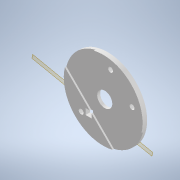
# Autodesk Inventor part: Matchboxscope_sample_v0
Saved by Autodesk Inventor 2022 (Build 260153000, 153)
## iProperties
Created: 2022-03-21
Part Number: Matchboxscope_sample_v0
Material: Generic
Document SubType Name: Modeling
Designer: Prakash Lab
Density: 1 g/cm^3
Appearance: Default
Author: Prakash Lab
Autodesk Inventor part; units mm, degrees
ref_plane "YZ Plane" through (0, 0, 0) normal (1, 0, 0) x (0, 1, 0)
ref_plane "XZ Plane" through (0, 0, 0) normal (0, 1, 0) x (-1, 0, 0)
ref_plane "XY Plane" through (0, 0, 0) normal (0, 0, 1) x (1, 0, 0)
ref_plane "Work Plane1" through (0, 0, 0) normal (0, 0, 1) x (0.9792327, -0.2027397, 0)
sketch "Sketch1" plane through (0, 0, 0) normal (0, 0, 1) x (0.9792327, -0.2027397, 0)
  circle A0 centre (8.0687, 11.3576) radius 25.9979 projected
  circle A1 centre (8.0703, 11.3562) radius 3.8103 projected
  circle A2 centre (8.0703, 11.3562) radius 5
  point P0 (0, 0)
  dimension "d0" = 10
  constraints: 1 centre point, 1 coincident
  measures "d0" diameter of A2
extrude "Extrusion1" add sketch "Sketch1" along normal blind 4 contours A0
sketch "Sketch2" plane through (10.2037, 9.4859, 4) normal (0, 0, 1) x (1, 0, 0)
  line L0 (-10.2037, 54.0449) -> (-10.2037, -50.593) projected
  line L1 (-54.0467, -9.4859) -> (50.5907, -9.4859) projected
  line L2 (-15.9479, -15.1669) -> (4.4725, 20.2023)
  line L3 (4.4725, 20.2023) -> (19.4213, 5.2535)
  line L4 (19.4213, 5.2535) -> (-15.9479, -15.1669)
  line L5 (-39.0985, 39.0967) -> (35.6425, -35.6447)
  line L6 (-0.781, 0) -> (9.2905, 10.0715)
  line L7 (-0.781, 0) -> (13.4622, 0) construction
  line L8 (-15.9479, -15.1669) -> (-0.781, 0)
  circle A0 centre (4.4725, 20.2023) radius 1.6
  circle A1 centre (19.4213, 5.2535) radius 1.6
  circle A2 centre (-15.9479, -15.1669) radius 1.6
  dimension "d17" = 18
  dimension "d18" = 22
  dimension "d19" = 30
  dimension "d20" = 45
  dimension "d21" = 15
  dimension "d22" = 3.2
  dimension "d23" = 3.2
  dimension "d24" = 3.2
  constraints: 14 end point, 3 centre point, 3 coincident, 1 collinear, 1 equal length, 1 horizontal, 1 parallel, 3 other
  measures "d17" distance from line of L6.start L3
  measures "d18" distance from line of L5 L2.start
  measures "d19" angle of L2 L4
  measures "d20" angle of L7 L6
  measures "d21" angle of L2 L6
  measures "d22" diameter of A0
  measures "d23" diameter of A1
  measures "d24" diameter of A2
extrude "Extrusion2" cut sketch "Sketch2" against normal through all contours A0 L3 L2 | L2 L3 A0 | A2 L8 L2 | L2 L4 A2 | A2 L4 L8 | A1 L4 L3 | L3 L4 A1
sketch "Sketch3" plane through (10.2037, 9.4859, 4) normal (0, 0, 1) x (1, 0, 0)
  line L0 (-35.7047, 22.4019) -> (13.1872, -35.1292) projected
  line L1 (32.542, -18.6808) -> (-16.3499, 38.8503) projected
  line L2 (40.2702, -21.1784) -> (-21.1782, 40.2703)
  line L3 (-21.1782, 40.2703) -> (-40.2702, 21.1784)
  line L4 (-40.2702, 21.1784) -> (21.1782, -40.2703)
  line L5 (21.1782, -40.2703) -> (40.2702, -21.1784)
  line L6 (40.2702, -21.1784) -> (-40.2702, 21.1784) construction
  line L7 (-21.1782, 40.2703) -> (21.1782, -40.2703) construction
  point P0 (0, 0)
  dimension "d16" = 27
  constraints: 12 end point, 2 midpoint, 2 parallel, 1 perpendicular
  measures "d16" distance of L3.end L2.end
extrude "Extrusion3" cut sketch "Sketch3" against normal blind 1
sketch "Sketch4" plane through (0, 0, 4) normal (0, 0, 1) x (0.9792327, -0.2027397, 0)
  circle A0 centre (-11.3769, -5.9318) radius 1.02 projected
  line L0 (-17.8452, -14.9951) -> (20.0302, -11.9207) projected
  line L1 (-7.3769, -9.6034) -> (-11.3769, -9.6034)
  line L2 (-11.3769, -9.6034) -> (-11.3769, -13.6034)
  line L3 (-11.3769, -13.6034) -> (-7.3769, -13.6034)
  line L4 (-7.3769, -13.6034) -> (-7.3769, -9.6034)
  line L5 (-7.3769, -9.6034) -> (-11.3769, -13.6034) construction
  line L6 (-11.3769, -9.6034) -> (-7.3769, -13.6034) construction
  circle A1 centre (-2.4923, 4.0739) radius 1 projected
  line L7 (-7.7982, -5.7154) -> (29.4127, 1.9886) projected
  line L8 (-1.2714, -1.0289) -> (2.6455, -0.218)
  line L9 (2.6455, -0.218) -> (3.4565, -4.1349)
  line L10 (3.4565, -4.1349) -> (-0.4605, -4.9459)
  line L11 (-0.4605, -4.9459) -> (-1.2714, -1.0289)
  line L12 (-1.2714, -1.0289) -> (3.4565, -4.1349) construction
  line L13 (2.6455, -0.218) -> (-0.4605, -4.9459) construction
  line L14 (-1.2714, -1.0289) -> (2.7286, -1.0289) construction
  point P0 (0, 0)
  point P1 (-9.3769, -11.6034)
  point P2 (1.0925, -2.5819)
  dimension "d25" = 2
  dimension "d28" = 4
  dimension "d29" = 4
  dimension "d30" = 4
  dimension "d31" = 11.697
  dimension "d32" = 4
  constraints: 26 end point, 5 parallel, 4 midpoint, 2 horizontal, 2 perpendicular, 1 equal length
  measures "d25" horizontal distance of point (-9.377, -11.603) A0.centre
  measures "d28" distance between parallel lines of L2 L4
  measures "d29" distance between parallel lines of L3 L1
  measures "d30" distance of L8.start L8.end
  measures "d31" angle of L14 L8
  measures "d32" distance of L8.end L9.end
extrude "Extrusion4" cut sketch "Sketch4" against normal blind 25.4 contours L4 L3 L2 L1 | L11 L8 L9 L7 | L7 L9 L10 L11
sketch "Sketch5" plane through (0, 0, 4) normal (0, 0, 1) x (0.9792327, -0.2027397, 0)
  circle A0 centre (-4.4731, -6.7275) radius 1.6 projected
  line L0 (2.8886, -1.3919) -> (3.4565, -4.1349) projected
  line L1 (3.4565, -4.1349) -> (-0.4605, -4.9459) projected
  line L2 (-0.4605, -4.9459) -> (-1.2714, -1.0289) projected
  line L3 (-1.2714, -1.0289) -> (1.4716, -0.461) projected
  line L4 (1.4716, -0.461) -> (-17.9131, 12.2738) projected
  arc A1 (-17.9131, 12.2738) -> (19.2256, -12.1245) centre (8.0687, 11.3576) ccw projected
  line L5 (19.2256, -12.1245) -> (2.8886, -1.3919) projected
  circle A2 centre (1.9035, -6.4989) radius 0.9
  circle A3 centre (-2.8244, -3.3929) radius 0.9
  point P0 (0, 0)
  dimension "d33" = 1.8
  dimension "d34" = 1.8
  dimension "d35" = 2
  dimension "d36" = 2
  constraints: 2 centre point
  measures "d33" diameter of A2
  measures "d34" diameter of A3
  measures "d35" distance from line of A3.centre L2
  measures "d36" distance from line of L1 A2.centre
extrude "Extrusion5" cut sketch "Sketch5" against normal blind 4 contours A2 | A3
body "Solid1"
